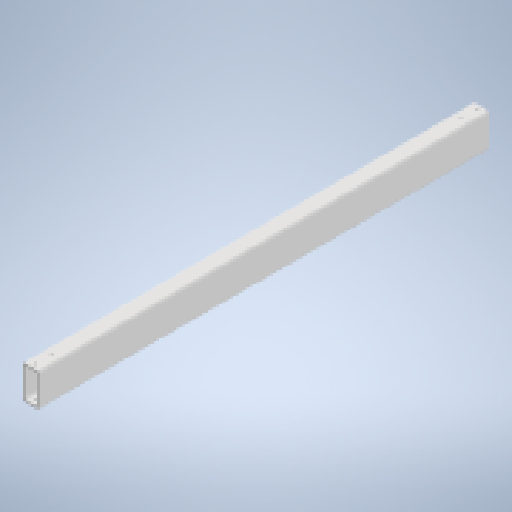
# Autodesk Inventor part: 2x4_Tube
Saved by Autodesk Inventor 2023 (Build 270158000, 158)
## iProperties
Created: 2022-05-07
Part Number: 2x4_Tube
Material: Generic
Document SubType Name: Modeling
Designer: plebbb
Density: 1 g/cm^3
Appearance: Default
Mass: 2205.6 g
Surface Area: 6723.67 cm^2
Volume: 2205.6 cm^3
Author: plebbb
Autodesk Inventor part; units mm, degrees
ref_plane "YZ Plane" through (0, 0, 0) normal (1, 0, 0) x (0, 1, 0)
ref_plane "XZ Plane" through (0, 0, 0) normal (0, 1, 0) x (-1, 0, 0)
ref_plane "XY Plane" through (0, 0, 0) normal (0, 0, 1) x (1, 0, 0)
sketch "Sketch1" plane through (0, 0, 0) normal (0, 0, 1) x (1, 0, 0)
  line L0 (0, 0) -> (50.8, 0)
  line L1 (50.8, 0) -> (50.8, 101.6)
  line L2 (50.8, 101.6) -> (0, 101.6)
  line L3 (0, 101.6) -> (0, 0)
  dimension "d0" = 101.6
  dimension "d1" = 50.8
  constraints: 8 end point, 2 parallel, 1 horizontal, 1 perpendicular
  measures "d0" distance of L0.end L1.end
  measures "d1" distance of L0.start L0.end
extrude "Extrusion1" add sketch "Sketch1" along normal blind 1320.8
shell "Shell1" thickness 6.35 removed faces 2 at (16.9333, 67.7333, 1320.8) at (16.9333, 67.7333, 0)
fillet "Fillet1" radius 6.35 8 edges at (6.35, 95.25, 660.4) (6.35, 6.35, 660.4) (44.45, 6.35, 660.4) (44.45, 95.25, 660.4) (50.8, 101.6, 660.4) (50.8, 0, 660.4) (0, 0, 660.4) (0, 101.6, 660.4)
sketch "Sketch2" plane through (6.35, 0, 0) normal (0, -1, 0) x (1, 0, 0)
  circle A0 centre (19.05, 63.1) radius 4
  circle A1 centre (19.05, 13.1) radius 4
  line L0 (19.05, 63.1) -> (19.05, 13.1) construction
  line L1 (0, 0) -> (38.1, 0) construction
  line L2 (38.1, 1320.8) -> (38.1, 0) construction
  line L3 (38.1, 660.4) -> (-101.1432, 660.4) construction
  circle A2 centre (19.05, 1257.7) radius 4
  circle A3 centre (19.05, 1307.7) radius 4
  point P0 (-6.35, 0)
  point P1 (19.05, 38.1)
  point P2 (19.05, 0)
  dimension "d6" = 8
  dimension "d7" = 38.1
  dimension "d8" = 50
  constraints: 4 centre point, 4 end point, 3 midpoint, 2 symmetric about line, 1 equal radius, 1 perpendicular, 1 vertical, 1 vertical alignment, 2 other
  measures "d6" diameter of A0
  measures "d7" vertical distance of point (-6.35, 0) point (19.05, 38.1)
  measures "d8" distance of L0.start L0.end
extrude "Extrusion2" cut sketch "Sketch2" against normal blind 1244.6
body "Solid1"
